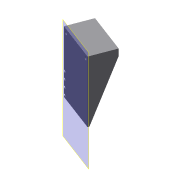
# Autodesk Inventor part: USSensor Backing
Saved by Autodesk Inventor 2018 (Build 220112000, 112)
## iProperties
Created: 2018-10-19
Part Number: USSensor Backing
Material: Generic
Document SubType Name: Modeling
Designer: Vulnic
Density: 1 g/cm^3
Appearance: Default
Author: Vulnic
Autodesk Inventor part; units mm, degrees
ref_plane "YZ Plane" through (0, 0, 0) normal (1, 0, 0) x (0, 1, 0)
ref_plane "XZ Plane" through (0, 0, 0) normal (0, 1, 0) x (-1, 0, 0)
ref_plane "XY Plane" through (0, 0, 0) normal (0, 0, 1) x (1, 0, 0)
ref_plane "Work Plane1" through (12.7619, -1.356, 21.3175) normal (0.3543575, 0, -0.93511) x (0, -1, 0)
sketch "Sketch1" plane through (12.7619, -1.356, 21.3175) normal (0.3543575, 0, -0.93511) x (0, -1, 0)
  line L0 (-22.86, -10.16) -> (-22.86, 10.16) projected
  line L1 (7.62, -10.16) -> (-22.86, -10.16)
  line L2 (-22.86, 10.16) -> (22.86, 10.16) projected
  line L3 (0.1143, 9.0805) -> (0.1143, 9.9695) projected
  line L4 (-0.7747, 9.0805) -> (0.1143, 9.0805) projected
  line L5 (-0.7747, 9.9695) -> (-0.7747, 9.0805) projected
  line L6 (0.1143, 9.9695) -> (-0.7747, 9.9695) projected
  line L7 (6.9723, 9.0805) -> (6.9723, 9.9695) projected
  line L8 (6.0833, 9.0805) -> (6.9723, 9.0805) projected
  line L9 (6.0833, 9.9695) -> (6.0833, 9.0805) projected
  line L10 (6.9723, 9.9695) -> (6.0833, 9.9695) projected
  line L11 (3.5433, 9.0805) -> (3.5433, 9.9695) projected
  line L12 (2.6543, 9.0805) -> (3.5433, 9.0805) projected
  line L13 (2.6543, 9.9695) -> (2.6543, 9.0805) projected
  line L14 (3.5433, 9.9695) -> (2.6543, 9.9695) projected
  line L15 (-3.3147, 9.0805) -> (-3.3147, 9.9695) projected
  line L16 (-4.2037, 9.0805) -> (-3.3147, 9.0805) projected
  line L17 (-4.2037, 9.9695) -> (-4.2037, 9.0805) projected
  line L18 (-3.3147, 9.9695) -> (-4.2037, 9.9695) projected
  circle A0 centre (21.0344, 8.4074) radius 0.7937 projected
  circle A1 centre (21.0344, -8.4074) radius 0.7937 projected
  circle A2 centre (-21.0344, 8.4074) radius 0.7937 projected
  circle A3 centre (-21.0344, -8.4074) radius 0.7937 projected
  line L19 (-4.2037, 9.9695) -> (-4.2037, 10.16)
  line L20 (-3.3147, 9.9695) -> (-3.3147, 10.16)
  line L21 (-0.7747, 9.9695) -> (-0.7747, 10.16)
  line L22 (0.1143, 9.9695) -> (0.1143, 10.16)
  line L23 (2.6543, 9.9695) -> (2.6543, 10.16)
  line L24 (3.5433, 9.9695) -> (3.5433, 10.16)
  line L25 (-22.86, -10.16) -> (7.62, -10.16)
  line L26 (7.62, -10.16) -> (7.62, 10.16)
  point P0 (-1.356, 19.4878)
  dimension "d0" = 30.48
  constraints: 18 end point, 5 vertical, 1 parallel, 1 point on line, 8 other
  measures "d0" distance of L1.start L0.start
extrude "Extrusion1" add sketch "Sketch1" along normal blind 12 contours L0 L2 L19 L17 L16 L15 L20 L21 L5 L4 L3 L22 L23 L13 L12 L11 L24 L26 L1
sketch "Sketch2" plane through (17.0142, -1.356, 10.0962) normal (0.3543575, 0, -0.93511) x (-0.93511, 0, -0.3543575)
  line L0 (9.9695, -6.0833) -> (10.1821, -6.0833)
  line L1 (10.1821, -6.0833) -> (10.1821, -6.9734)
  line L2 (10.1821, -6.9734) -> (9.9695, -6.9734)
  line L3 (9.9695, -6.9734) -> (9.9695, -6.0833)
  point P0 (19.4878, 1.356)
  constraints: 8 end point, 2 parallel, 1 horizontal, 1 perpendicular
extrude "Extrusion2" cut sketch "Sketch2" against normal through all
sketch "Sketch3" plane through (3.2612, 2.8477, 17.7172) normal (-0.93511, 0, -0.3543575) x (-0.3543575, 0, 0.93511)
  line L0 (-12, 0) -> (-12, 18.6563) projected
  line L1 (-12, 15.3816) -> (-0.6665, -11.8237)
  line L2 (0, -11.8237) -> (-12, -11.8237) projected
  line L3 (-0.6665, -11.8237) -> (-12, -11.8237)
  line L4 (-12, -11.8237) -> (-12, 15.3816)
  point P0 (-15.4119, -2.8477)
  constraints: 6 end point, 1 collinear, 1 perpendicular, 1 point on line
extrude "Extrusion3" cut sketch "Sketch3" against normal through all
body "Solid1"
